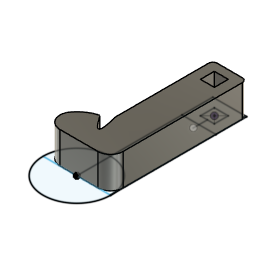
CTS Rubber Band Launcher (Autodesk Fusion 360 design; units mm, degrees)
Autodesk Fusion 360 part; units mm, degrees
sketch "Sketch1" plane through (0, 0, 0) normal (0, 0, 1) x (1, 0, 0)
  line L0 (1.651, -1.651) -> (-1.651, -1.651)
  line L1 (-1.651, -1.651) -> (-1.651, 1.651)
  line L2 (-1.651, 1.651) -> (1.651, 1.651)
  line L3 (1.651, 1.651) -> (1.651, -1.651)
  line L4 (1.651, -1.651) -> (-1.651, 1.651) construction
  line L5 (-1.651, -1.651) -> (1.651, 1.651) construction
  line L6 (0, -1.651) -> (0, -5)
  line L7 (4, -3.651) -> (4, -28.651)
  line L8 (-4, -3.651) -> (-4, -28.651)
  circle A0 centre (-4, -28.651) radius 8
  line L9 (-4, -3.651) -> (4, -3.651)
  line L10 (4, -3.651) -> (4, 3.651)
  line L11 (4, 3.651) -> (-4, 3.651)
  line L12 (-4, 3.651) -> (-4, -3.651)
  line L13 (4, -28.651) -> (-12, -28.651)
  dimension "d1" = 3.302
  dimension "d3" = 4
  dimension "d4" = 4
  dimension "d5" = 25
  dimension "d6" = 25
  dimension "d7" = 2
  dimension "d8" = 2
  dimension "d19" = 3.302
  constraint horizontal L0
  constraint perpendicular L0 L1
  constraint parallel L0 L2
  constraint parallel L1 L3
  constraint coincident L4 origin
  constraint coincident L5 origin
  constraint midpoint L0 L6.start
  constraint perpendicular L0 L6
  constraint vertical L8
  constraint coincident L8.end A0.centre
  constraint coincident L7.end A0
  constraint perpendicular L7 L9
  constraint perpendicular L9 L10
  constraint perpendicular L10 L11
  constraint perpendicular L9 L12
  constraint coincident A0 L13.end
  measures "d1" distance of L1.end L2.end
  measures "d3" distance of L6 L8
  measures "d4" distance of L6 L7
  measures "d5" distance of L7.start L7.end
  measures "d6" distance of L8.start L8.end
  measures "d7" distance of L0 L9
  measures "d8" distance of L2 L11
  measures "d19" distance of L0.end L1.end
extrude "Extrude1" add sketch "Sketch1" along normal blind 7.5 contours L7 L8 A0 L9 | L9 L10 L11 L12 | L8 A0 L13 | L8 A0 L13
fillet "Fillet1" radius 3 2 edges at (4, -28.651, 3.75) (-12, -28.651, 3.75)
fillet "Fillet2" radius 1 2 edges at (4, 3.651, 3.75) (-4, 3.651, 3.75)
sketch "Sketch2" plane through (0, 0, 7.5) normal (0, 0, 1) x (-1, 0, 0)
  line L0 (1.651, -1.651) -> (-1.651, -1.651)
  line L1 (-1.651, -1.651) -> (-1.651, 1.651)
  line L2 (-1.651, 1.651) -> (1.651, 1.651)
  line L3 (1.651, 1.651) -> (1.651, -1.651)
  arc A0 (3, -3.651) -> (4, -2.651) centre (3, -2.651) ccw
  line L4 (4, -2.651) -> (4, 20.651)
  arc A1 (4, 20.651) -> (10.4, 23.851) centre (4, 28.651) ccw
  arc A2 (10.4, 23.851) -> (8, 28.651) centre (8, 25.651) ccw
  line L5 (8, 28.651) -> (-1, 28.651)
  arc A3 (-1, 28.651) -> (-4, 25.651) centre (-1, 25.651) ccw
  line L6 (-4, 25.651) -> (-4, -2.651)
  arc A4 (-4, -2.651) -> (-3, -3.651) centre (-3, -2.651) ccw
  line L7 (-3, -3.651) -> (3, -3.651)
  spline S0 degree 5 poles (5, 16) (4.8292, 16.5616) (4.5076, 17.6395) (4.0852, 19.1209) (3.6439, 20.8204) (3.3095, 22.454) (3.2122, 23.5517) (3.3723, 24.0679) (3.8023, 23.9742) (4.4935, 23.2901) (5.4271, 22.0585) (6.3522, 20.6701) (7.1402, 19.4163) (7.7065, 18.4876) (8, 18) knots 0 0 0 0 0 0 0.1 0.2 0.3 0.4 0.5 0.6 0.7 0.8 0.9 1 1 1 1 1 1
  line L8 (4, 19.4919) -> (6.0828, 21.0539)
  point P0 (3.4661, 23.9318)
  constraint coincident S0 L8.start
  constraint coincident L4 L8.start
  constraint coincident S0 L8.end
  constraint coincident A1 L8.end
extrude "Extrude2" cut sketch "Sketch2" against normal blind 10 contours L4 A1 S0 L8 | A1 S0 L8
fillet "Fillet3" radius 0.5 2 edges at (-4, -19.4919, 3.75) (-6.154, -20.9464, 3.75)
